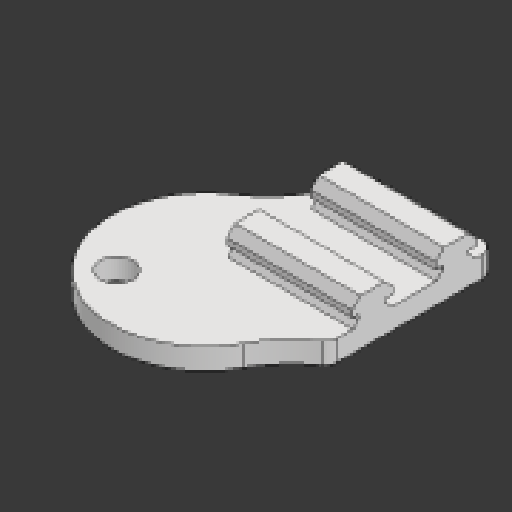
# Autodesk Inventor part: Webcam Mount
Saved by Autodesk Inventor 2023 (Build 270158000, 158)
## iProperties
Created: 2023-01-08
Part Number: Webcam Mount
Material: Generic
Document SubType Name: Modeling
Designer: alber
Density: 1 g/cm^3
Appearance: Default
Author: alber
Autodesk Inventor part; units mm, degrees
ref_plane "YZ Plane" through (0, 0, 0) normal (1, 0, 0) x (0, 1, 0)
ref_plane "XZ Plane" through (0, 0, 0) normal (0, 1, 0) x (-1, 0, 0)
ref_plane "XY Plane" through (0, 0, 0) normal (0, 0, 1) x (1, 0, 0)
sketch "Sketch1" plane through (0, 0, 0) normal (1, 0, 0) x (0, 1, 0)
  line L0 (-10.3707, -4.7464) -> (-8.7536, -3.1293)
  line L1 (-10.3707, 15.395) -> (-8.7381, 17.0275)
  arc A0 (-7.8549, 16.6) -> (-8.7381, 17.0275) centre (-8.4, 16.6) ccw
  line L2 (-7.8549, 16.6) -> (-7.8549, 15.135)
  line L3 (-7.8549, 15.135) -> (-6.3429, 15.135)
  line L4 (-6.3429, 15.135) -> (-4.3451, 17.1329)
  line L5 (-4.3451, 17.1329) -> (-4.3451, 22.8671)
  line L6 (-4.3451, 22.8671) -> (-6.3429, 24.865)
  line L7 (-6.3429, 24.865) -> (-7.8549, 24.865)
  line L8 (-7.8549, 24.865) -> (-7.8549, 23.8568)
  arc A1 (-9.0499, 23.3618) -> (-7.8549, 23.8568) centre (-8.5549, 23.8568) ccw
  line L9 (-9.0499, 23.3618) -> (-10.3707, 24.6827)
  line L10 (-10.3707, 24.6827) -> (-10.3707, 30.0707)
  line L11 (-10.3707, 30.0707) -> (-11.3707, 30.0707)
  line L12 (-11.9747, -9.2902) -> (-10.3707, -9.2902)
  arc A2 (-7.9, -3.4828) -> (-8.7536, -3.1293) centre (-8.4, -3.4828) ccw
  line L13 (-7.9, -3.4828) -> (-7.9, -4.9101)
  line L14 (-7.9, -4.9101) -> (-6.3243, -4.9101)
  line L15 (-6.3243, -4.9101) -> (-4.3, -2.8858)
  line L16 (-4.3, -2.8858) -> (-4.3, 2.8858)
  line L17 (-4.3, 2.8858) -> (-6.3243, 4.9101)
  line L18 (-6.3243, 4.9101) -> (-7.9, 4.9101)
  line L19 (-7.9, 4.9101) -> (-7.9, 3.4828)
  arc A3 (-8.7536, 3.1293) -> (-7.9, 3.4828) centre (-8.4, 3.4828) ccw
  line L20 (-8.7536, 3.1293) -> (-10.3707, 4.7464)
  line L21 (-10.3707, 15.395) -> (-10.3707, 4.7464)
  line L22 (-10.3707, 30.0707) -> (-15.3707, 30.0707)
  line L23 (-15.3707, 30.0707) -> (-15.3707, -9.2902)
  line L24 (-15.3707, -9.2902) -> (-10.3707, -9.2902)
  line L25 (-10.3707, 24.6827) -> (-10.3707, 30.0707)
  line L26 (-10.3707, -9.2902) -> (-10.3707, -4.7464)
  line L27 (-10.3707, 4.7464) -> (-10.3707, 15.395)
  point P0 (0, 0)
  point P1 (-7.8549, 16.6)
  point P2 (-9.0499, 23.3618)
  dimension "d0" = 5
  constraints: 56 end point, 8 point on circle, 4 centre point, 4 parallel, 1 horizontal, 1 perpendicular, 1 point on line
  measures "d0" distance of L12.end L23.end
extrude "Extrusion1" add sketch "Sketch1" against normal blind 30
sketch "Sketch2" plane through (0, -15.3707, -9.2902) normal (0, -1, 0) x (1, 0, 0)
  line L0 (-30, 0) -> (-30, 39.3609) projected
  circle A0 centre (-30, 39.3609) radius 22.5
  circle A1 centre (-40.6066, 49.9675) radius 4
  point P0 (0, 9.2902)
  dimension "d3" = 45
  dimension "d4" = 8
  dimension "d5" = 10.6066
  dimension "d6" = 10.6066
  constraints: 2 centre point
  measures "d3" diameter of A0
  measures "d4" diameter of A1
  measures "d5" horizontal distance of A1.centre L0.end
  measures "d6" horizontal distance of A1.centre L0.end
extrude "Extrusion2" add sketch "Sketch2" against normal blind 5
fillet "Fillet1" radius 30 1 edges at (-7.5, -12.8707, 30.0707)
fillet "Fillet2" radius 3 1 edges at (0, -12.8707, 30.0707)
sketch "Sketch3" plane through (-30, 0, 0) normal (-1, 0, 0) x (0, 0, 1)
  line L0 (7.5707, -15.3707) -> (7.5707, -10.3707) projected
  line L1 (-9.2902, -10.3707) -> (-9.2902, -15.3707) projected
  line L2 (7.5707, -15.3707) -> (-9.2902, -15.3707)
  line L3 (-9.2902, -15.3707) -> (-9.2902, -10.3707)
  line L4 (-9.2902, -10.3707) -> (7.5707, -10.3707)
  line L5 (7.5707, -10.3707) -> (7.5707, -15.3707)
  point P0 (0, 0)
  constraints: 8 end point, 2 parallel, 1 horizontal, 1 perpendicular
extrude "Extrusion3" cut sketch "Sketch3" against normal blind 0.75
fillet "Fillet3" radius 30 1 edges at (-29.25, -12.8707, 7.5707)
fillet "Fillet4" radius 3 1 edges at (0, -12.8707, -9.2902)
fillet "Fillet5" radius 3 1 edges at (-29.25, -12.8707, -9.2902)
equation "\"d6\" = d5"
body "Solid1"
